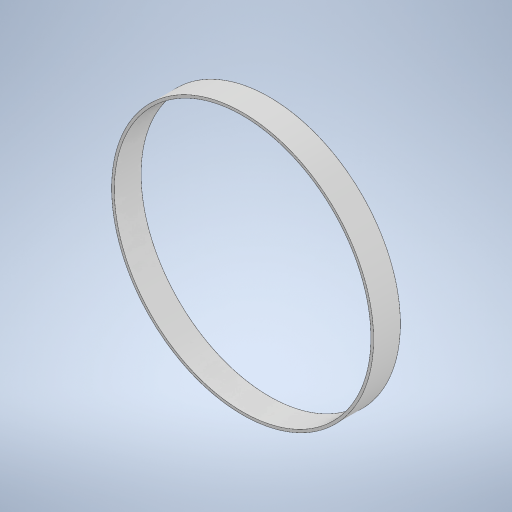
# Autodesk Inventor part: Connection_thing
Saved by Autodesk Inventor 2024.2 (Build 282272000, 272)
## iProperties
Created: 2024-01-17
Part Number: Connection_thing
Material: Generic
Document SubType Name: Modeling
Designer: filip
Density: 1 g/cm^3
Appearance: Default
Author: filip
Autodesk Inventor part; units mm, degrees
ref_plane "YZ Plane" through (0, 0, 0) normal (1, 0, 0) x (0, 1, 0)
ref_plane "XZ Plane" through (0, 0, 0) normal (0, 1, 0) x (-1, 0, 0)
ref_plane "XY Plane" through (0, 0, 0) normal (0, 0, 1) x (1, 0, 0)
sketch "Sketch1" plane through (0, 0, 0) normal (0, 0, 1) x (1, 0, 0)
  circle A0 centre (0, 0) radius 48.9
  circle A1 centre (0, 0) radius 47.9
  dimension "d0" = 97.8
  dimension "d1" = 1
  constraints: 2 centre point, 2 coincident
  measures "d0" diameter of A0
  measures "d1" radial gap between concentric circles of A0 A1
extrude "Extrusion1" add sketch "Sketch1" along normal blind 10
body "Solid1"
